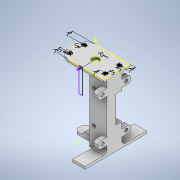
# Autodesk Inventor part: Gravitational viscometer P1
Saved by Autodesk Inventor 2020 (Build 240168000, 168)
## iProperties
Created: 2023-07-24
Part Number: Gravitational viscometer P1
Material: Generic
Document SubType Name: Modeling
Designer: 56992
Density: 1 g/cm^3
Appearance: Default
Author: 56992
Autodesk Inventor part; units mm, degrees
ref_plane "YZ Plane" through (0, 0, 0) normal (1, 0, 0) x (0, 1, 0)
ref_plane "XZ Plane" through (0, 0, 0) normal (0, 1, 0) x (-1, 0, 0)
ref_plane "XY Plane" through (0, 0, 0) normal (0, 0, 1) x (1, 0, 0)
sketch "Sketch1" plane through (0, 0, 0) normal (0, 0, 1) x (1, 0, 0)
  line L0 (0, 0) -> (30, 0)
  line L1 (30, 0) -> (30, 90)
  line L2 (30, 90) -> (0, 90)
  line L3 (0, 90) -> (0, 0)
  dimension "d0" = 90
  dimension "d1" = 30
  constraints: 8 end point, 2 parallel, 1 horizontal, 1 perpendicular
  measures "d0" distance between parallel lines of L0 L2
  measures "d1" distance between parallel lines of L3 L1
extrude "Extrusion1" add sketch "Sketch1" along normal blind 12
sketch "Sketch2" plane through (0, 90, 0) normal (0, 1, 0) x (1, 0, 0)
  circle A0 centre (6, -6) radius 3.9
  line L0 (30, 0) -> (0, 0) projected
  line L1 (0, 0) -> (0, -12) projected
  dimension "d4" = 7.8
  dimension "d5" = 6
  dimension "d6" = 6
  constraints: 1 centre point
  measures "d4" diameter of A0
  measures "d5" distance from line of L0 A0.centre
  measures "d6" distance from line of L1 A0.centre
extrude "Extrusion2" cut sketch "Sketch2" against normal blind 120
sketch "Sketch3" plane through (0, 0, 12) normal (0, 0, 1) x (1, 0, 0)
  line L0 (0, 90) -> (0, 0) projected
  line L1 (0, 83) -> (12, 83)
  line L2 (12, 83) -> (12, 7)
  line L3 (12, 7) -> (0, 7)
  line L4 (0, 7) -> (0, 83)
  line L5 (30, 90) -> (0, 90) projected
  line L6 (0, 0) -> (30, 0) projected
  point P0 (0, 7)
  dimension "d9" = 7
  dimension "d10" = 7
  dimension "d11" = 12
  constraints: 8 end point, 2 parallel, 1 horizontal, 1 perpendicular, 1 point on line
  measures "d9" distance between parallel lines of L5 L1
  measures "d10" distance between parallel lines of L6 L3
  measures "d11" distance between parallel lines of L0 L2
extrude "Extrusion3" cut sketch "Sketch3" against normal blind 120
sketch "Sketch4" plane through (0, 0, 0) normal (0, -1, 0) x (1, 0, 0)
  line L0 (30, 0) -> (30, 12) projected
  line L1 (30, 0) -> (0, 0)
  line L2 (0, 0) -> (0, -12)
  line L3 (0, -12) -> (30, -12)
  line L4 (30, -12) -> (30, 0)
  line L5 (0, 0) -> (0, 12) projected
  dimension "d14" = 0
  dimension "d15" = 12
  constraints: 8 end point, 2 parallel, 1 horizontal, 1 perpendicular
  measures "d14" distance between parallel lines of L5 L2
  measures "d15" distance between parallel lines of L1 L3
extrude "Extrusion4" add sketch "Sketch4" against normal blind 3
sketch "Sketch5" plane through (30, 90, 12) normal (0, 1, 0) x (1, 0, 0)
  point P0 (-30, 12)
sketch "Sketch6" plane through (0, 90, 0) normal (0, 1, 0) x (1, 0, 0)
  point P0 (0, 0)
sketch "Sketch7" plane through (30, 90, 12) normal (0, 1, 0) x (1, 0, 0)
  line L0 (-30, 0) -> (0, 0) projected
  line L1 (-30, 24) -> (-30, 0) projected
  line L2 (-10, 0) -> (-30, 0)
  line L3 (-30, 0) -> (-30, 24)
  line L4 (-30, 24) -> (-10, 24)
  line L5 (-10, 24) -> (-10, 0)
  circle A0 centre (-24, 6) radius 4.25 projected
  circle A1 centre (-24, 6) radius 3.75
  point P0 (-30, 12)
  point P1 (-25, 0)
  point P2 (-30, 5)
  point P3 (-30, 5)
  point P4 (-25, 0)
  dimension "d22" = 20
  dimension "d23" = 7.5
  constraints: 8 end point, 2 parallel, 1 centre point, 1 coincident, 1 horizontal, 1 perpendicular, 1 point on line
  measures "d22" distance between parallel lines of L1 L5
  measures "d23" diameter of A1
extrude "Extrusion5" add sketch "Sketch7" along normal blind 2 contours L1 L4 L5 L0 | A0
fillet "Fillet7" radius 0.5 4 edges at (2.25, 92, 6) (2.1, 83, 6) (2.1, 7, 6) (2.1, 0, 6)
chamfer "Chamfer2" distance 3 angle 45 1 edges at (10, 90, 0)
chamfer "Chamfer3" distance 3 angle 45 1 edges at (15, 3, 0)
chamfer "Chamfer4" [suppressed]
sketch "Sketch8" plane through (30, 92, 12) normal (0, 1, 0) x (1, 0, 0)
  point P0 (-30, 12)
sketch "Sketch9" plane through (30, 92, 12) normal (0, 1, 0) x (1, 0, 0)
  point P0 (-30, 12)
sketch "Sketch10" plane through (30, 92, 12) normal (0, 1, 0) x (1, 0, 0)
  line L0 (0, 12) -> (0, 0) projected
  line L1 (0, 12) -> (-30, 12)
  line L2 (-30, 12) -> (-30, 24)
  line L3 (-30, 24) -> (0, 24)
  line L4 (0, 24) -> (0, 12)
  line L5 (-30, 24) -> (-30, 0) projected
  line L6 (-10, 24) -> (-30, 24) projected
  point P0 (-30, 12)
  dimension "d41" = 0
  dimension "d42" = 0
  constraints: 8 end point, 2 parallel, 1 horizontal, 1 perpendicular
  measures "d41" distance between parallel lines of L5 L2
  measures "d42" distance between parallel lines of L6 L3
extrude "Extrusion6" cut sketch "Sketch10" against normal blind 100
sketch "Sketch11" plane through (0, 0, 0) normal (0, 0, -1) x (-1, 0, 0)
  line L0 (-19, 74) -> (-5.5, 74)
  line L1 (-5.5, 74) -> (-5.5, 8)
  line L2 (-5.5, 8) -> (-19, 8)
  line L3 (-19, 8) -> (-19, 74)
  line L4 (-12, 83) -> (0, 83) projected
  circle A0 centre (-15.3, 60) radius 2.05
  circle A1 centre (-15.3, 23) radius 2.05
  point P0 (0, 0)
  point P1 (0, 92)
  point P2 (-10, 83)
  dimension "d45" = 13.5
  dimension "d46" = 66
  dimension "d47" = 5.5
  dimension "d48" = 9
  dimension "d49" = 37
  dimension "d50" = 14
  dimension "d51" = 3.7
  dimension "d52" = 3.7
  dimension "d53" = 4.1
  dimension "d54" = 4.1
  constraints: 8 end point, 2 centre point, 2 parallel, 1 horizontal, 1 perpendicular
  measures "d45" distance between parallel lines of L1 L3
  measures "d46" distance between parallel lines of L2 L0
  measures "d47" distance from line of point (0, 92) L1
  measures "d48" distance between parallel lines of L4 L0
  measures "d49" distance of A1.centre A0.centre
  measures "d50" distance from line of L0 A0.centre
  measures "d51" distance from line of L3 A0.centre
  measures "d52" distance from line of L3 A1.centre
  measures "d53" diameter of A0
  measures "d54" diameter of A1
sketch "Sketch12" plane through (0, 0, 0) normal (0, 0, -1) x (-1, 0, 0)
  point P0 (0, 0)
extrude "Extrusion7" cut sketch "Sketch11" against normal blind 100 contours A0 | A1
sketch "Sketch13" plane through (0, 0, 0) normal (0, 0, -1) x (-1, 0, 0)
  line L0 (-10, 7) -> (-12, 9) projected
  line L1 (-10, 7) -> (-12, 7)
  line L2 (-12, 7) -> (-12, 83)
  line L3 (-12, 83) -> (-10, 83)
  line L4 (-10, 83) -> (-10, 7)
  line L5 (-12, 83) -> (0, 83) projected
  point P0 (0, 0)
  point P1 (-10, 83)
  dimension "d57" = 2
  dimension "d58" = 0
  constraints: 8 end point, 2 parallel, 1 horizontal, 1 perpendicular
  measures "d57" distance between parallel lines of L4 L2
  measures "d58" distance between parallel lines of L5 L3
extrude "Extrusion8" add sketch "Sketch13" against normal blind 12 contours L0 L2 L3 L4
sketch "Sketch14" plane through (0, 0, 0) normal (0, 0, -1) x (-1, 0, 0)
  line L0 (-15.3, 56.8) -> (-30, 56.8)
  line L1 (-30, 56.8) -> (-30, 26.2)
  line L2 (-30, 26.2) -> (-15.3, 26.2)
  line L3 (-15.3, 26.2) -> (-15.3, 56.8)
  circle A0 centre (-15.3, 60) radius 2.05 projected
  circle A1 centre (-15.3, 23) radius 2.05 projected
  line L4 (-30, 0) -> (-30, 90) projected
  line L5 (-10, 83) -> (0, 83) projected
  line L6 (-10, 83) -> (-15.3, 83)
  line L7 (-15.3, 83) -> (-15.3, 64)
  line L8 (-15.3, 64) -> (-10, 64)
  line L9 (-10, 64) -> (-10, 83)
  line L10 (-12, 9) -> (-10, 7) projected
  line L11 (-10, 7) -> (-15.3, 7)
  line L12 (-15.3, 7) -> (-15.3, 19)
  line L13 (-15.3, 19) -> (-10, 19)
  line L14 (-10, 19) -> (-10, 7)
  point P0 (0, 0)
  dimension "d61" = 3.2
  dimension "d62" = 3.2
  dimension "d63" = 0
  dimension "d64" = 0
  dimension "d67" = 0
  dimension "d68" = 4
  dimension "d69" = 4
  constraints: 24 end point, 6 parallel, 3 horizontal, 3 perpendicular, 1 point on line
  measures "d61" distance from line of A0.centre L0
  measures "d62" distance from line of A1.centre L2
  measures "d63" distance from line of A0.centre L3
  measures "d64" distance between parallel lines of L4 L1
  measures "d67" distance from line of A0.centre L7
  measures "d68" distance from line of A1.centre L13
  measures "d69" distance from line of A0.centre L8
extrude "Extrusion9" cut sketch "Sketch14" against normal blind 7 contours L3 L2 L1 L0
sketch "Sketch15" plane through (0, 0, 0) normal (0, 0, -1) x (-1, 0, 0)
  point P0 (0, 0)
extrude "Extrusion10" cut sketch "Sketch14" against normal blind 4 contours L9 L8 L7 L6 | L11 L12 L13 L14
sketch "Sketch16" plane through (0, 0, 12) normal (0, 0, 1) x (1, 0, 0)
  line L0 (30, 0) -> (30, 90) projected
  line L1 (0, 0) -> (30, 0) projected
  line L2 (30, 90) -> (10, 90)
  line L3 (10, 90) -> (10, 0)
  line L4 (10, 0) -> (30, 0)
  line L5 (30, 0) -> (30, 90)
  line L6 (10, 83) -> (10, 7) projected
  circle A0 centre (15.3, 60) radius 2.05 projected
  circle A1 centre (15.3, 60) radius 2.15
  circle A2 centre (15.3, 23) radius 2.05 projected
  circle A3 centre (15.3, 23) radius 2.15
  dimension "d72" = 0
  dimension "d73" = 4.1
  dimension "d74" = 37
  dimension "d75" = 5.3
  dimension "d76" = 23
  constraints: 8 end point, 2 centre point, 2 coincident, 2 parallel, 1 horizontal, 1 perpendicular, 1 point on line
  measures "d72" distance between parallel lines of L6 L3
  measures "d73" diameter of A0
  measures "d74" distance of A2.centre A0.centre
  measures "d75" distance from line of L3 A2.centre
  measures "d76" distance from line of L1 A2.centre
extrude "Extrusion11" add sketch "Sketch16" along normal blind 5 contours L1 L3 L2 L0 | A1 | A3
sketch "Sketch17" plane through (0, 0, 0) normal (0, -1, 0) x (1, 0, 0)
  line L0 (10, 17) -> (30, 17) projected
  line L1 (30, 17) -> (16, 17)
  line L2 (16, 17) -> (16, -18)
  line L3 (16, -18) -> (30, -18)
  line L4 (30, -18) -> (30, 17)
  point P0 (0, 0)
  point P1 (16, 17)
  dimension "d79" = 35
  dimension "d80" = 14
  constraints: 8 end point, 2 parallel, 1 horizontal, 1 perpendicular
  measures "d79" distance between parallel lines of L0 L3
  measures "d80" distance between parallel lines of L4 L2
extrude "Extrusion12" add sketch "Sketch17" against normal blind 3
sketch "Sketch18" plane through (0, 0, 0) normal (0, -1, 0) x (1, 0, 0)
  line L0 (30, 17) -> (16, 17)
  line L1 (16, 17) -> (16, 32)
  line L2 (16, 32) -> (30, 32)
  line L3 (30, 32) -> (30, 17)
  line L4 (0, 12) -> (10, 12) projected
  line L5 (16, 0) -> (16, -18) projected
  point P0 (0, 0)
  dimension "d83" = 20
  dimension "d84" = 0
  constraints: 8 end point, 2 parallel, 1 horizontal, 1 perpendicular
  measures "d83" distance between parallel lines of L4 L2
  measures "d84" distance between parallel lines of L5 L1
extrude "Extrusion13" add sketch "Sketch18" against normal blind 3
chamfer "Chamfer5" [suppressed]
sketch "Sketch19" plane through (20, 90, 0) normal (0, 1, 0) x (1, 0, 0)
  line L0 (-10, -12) -> (-10, -17) projected
  line L1 (10, 0) -> (10, -17) projected
  line L2 (-10, -17) -> (10, -17)
  line L3 (10, -17) -> (10, 0)
  line L4 (10, 0) -> (-10, 0)
  line L5 (-10, 0) -> (-10, -17)
  point P0 (-20, 0)
  constraints: 8 end point, 2 parallel, 1 horizontal, 1 perpendicular
extrude "Extrusion14" add sketch "Sketch19" along normal blind 2
sketch "Sketch20" plane through (30, 92, 12) normal (0, 1, 0) x (1, 0, 0)
  point P0 (-30, 12)
sketch "Sketch21" plane through (0, 83, 0) normal (-1, 0, 0) x (0, 0, 1)
  line L0 (0, -26.2) -> (0, 9) projected
  line L1 (12, 0) -> (12, 9) projected
  line L2 (0, 9) -> (12, 9)
  line L3 (12, 9) -> (12, 5)
  line L4 (12, 5) -> (0, 5)
  line L5 (0, 5) -> (0, 9)
  point P0 (0, -83)
  point P1 (0, 5)
  dimension "d92" = 4
  constraints: 8 end point, 2 parallel, 1 horizontal, 1 perpendicular, 1 point on line
  measures "d92" distance between parallel lines of L2 L4
extrude "Extrusion15" add sketch "Sketch21" along normal blind 5
sketch "Sketch22" plane through (30, 92, 12) normal (0, 1, 0) x (1, 0, 0)
  line L0 (-20, -5) -> (0, -5) projected
  line L1 (-35, 12) -> (-35, 0) projected
  line L2 (-20, -5) -> (-35, -5)
  line L3 (-35, -5) -> (-35, 0)
  line L4 (-35, 0) -> (-20, 0)
  line L5 (-20, 0) -> (-20, -5)
  point P0 (-30, 12)
  constraints: 8 end point, 2 parallel, 1 horizontal, 1 perpendicular
extrude "Extrusion16" add sketch "Sketch22" against normal blind 4
sketch "Sketch25" plane through (-5, 83, 0) normal (-1, 0, 0) x (0, 0, 1)
  line L0 (17, 9) -> (0, 9) projected
  line L1 (17, -80) -> (17, 9) projected
  line L2 (0, 9) -> (17, 9)
  line L3 (17, 9) -> (17, 5)
  line L4 (17, 5) -> (0, 5)
  line L5 (0, 5) -> (0, 9)
  line L6 (0, 5) -> (17, 5) projected
  line L7 (-2, 8) -> (19, 8)
  line L8 (19, 8) -> (19, 6)
  line L9 (19, 6) -> (-2, 6)
  line L10 (-2, 6) -> (-2, 8)
  point P0 (0, -83)
  dimension "d107" = 0
  dimension "d108" = 2
  dimension "d109" = 2
  dimension "d110" = 2
  dimension "d111" = 1
  dimension "d112" = 1
  constraints: 16 end point, 4 parallel, 2 horizontal, 2 perpendicular, 1 point on line
  measures "d107" distance between parallel lines of L6 L4
  measures "d108" distance between parallel lines of L9 L7
  measures "d109" distance between parallel lines of L1 L8
  measures "d110" distance between parallel lines of L5 L10
  measures "d111" distance between parallel lines of L0 L7
  measures "d112" distance between parallel lines of L4 L9
extrude "Extrusion17" add sketch "Sketch25" against normal blind 35 contours L7 L8 L9 L1 | L1 L9 L5 L7 | L5 L9 L10 L7
sketch "Sketch26" plane through (30, 92, 12) normal (0, 1, 0) x (1, 0, 0)
  arc A0 (-20, 7.4361) -> (-20, 4.5639) centre (-24, 6) ccw projected
  circle A1 centre (-24, 6) radius 3.9
  point P0 (-30, 12)
  dimension "d115" = 7.8
  constraints: 1 centre point, 1 coincident
  measures "d115" diameter of A1
extrude "Extrusion18" cut sketch "Sketch26" against normal blind 35
sketch "Sketch27" plane through (0, 0, 0) normal (-1, 0, 0) x (0, 0, 1)
  line L0 (12, 7) -> (12, 0) projected
  line L1 (0, 0) -> (12, 0)
  line L2 (12, 0) -> (12, 3)
  line L3 (12, 3) -> (0, 3)
  line L4 (0, 3) -> (0, 0)
  dimension "d118" = 3
  constraints: 8 end point, 2 parallel, 1 horizontal, 1 perpendicular, 1 point on line
  measures "d118" distance between parallel lines of L1 L3
extrude "Extrusion19" add sketch "Sketch27" along normal blind 6
chamfer "Chamfer6" distance 2 angle 45 2 edges at (-6, 1.5, 12) (-6, 1.5, 0)
fillet "Fillet8" radius 4 2 edges at (23, 3, 0) (23, 3, 17)
chamfer "Chamfer7" distance 4 angle 45 1 edges at (0, 3, 6)
sketch "Sketch28" plane through (-5, 89, -2) normal (0, 0, -1) x (-1, 0, 0)
  line L0 (0, 3) -> (-35, 3) projected
  line L1 (-35, 3) -> (0, 3)
  line L2 (0, 3) -> (0, -3)
  line L3 (0, -3) -> (-35, -3)
  line L4 (-35, -3) -> (-35, 3)
  line L5 (-20.3, -6) -> (-5, -6) projected
  point P0 (-5, -89)
  dimension "d128" = 3
  dimension "d129" = 5
  constraints: 8 end point, 2 parallel, 1 horizontal, 1 perpendicular
  measures "d128" distance between parallel lines of L5 L3
  measures "d129" distance from line of L5.end L2
extrude "Extrusion20" cut sketch "Sketch28" against normal blind 30
fillet_without_effect "Fillet9"
sketch "Sketch29" plane through (0, 83, 0) normal (0, -1, 0) x (1, 0, 0)
  point P0 (0, 0)
sketch "Sketch30" plane through (0, 0, 0) normal (0, 0, -1) x (-1, 0, 0)
  line L0 (-30, 7) -> (-30, 86) projected
  line L1 (-30, 86) -> (0, 86)
  line L2 (0, 86) -> (0, 76)
  line L3 (0, 76) -> (-30, 76)
  line L4 (-30, 76) -> (-30, 86)
  line L5 (-15.3, 83) -> (0, 83) projected
  point P0 (0, 0)
  dimension "d133" = 7
  dimension "d134" = 30
  constraints: 8 end point, 2 parallel, 1 horizontal, 1 perpendicular
  measures "d133" distance between parallel lines of L5 L3
  measures "d134" distance between parallel lines of L0 L2
extrude "Extrusion21" cut sketch "Sketch30" against normal blind 30
sketch "Sketch31" plane through (15.3, 76, 0) normal (0, 1, 0) x (1, 0, 0)
  line L0 (-2.05, 0) -> (2.05, 0) projected
  line L1 (-15.3, -12) -> (-15.3, 0) projected
  line L2 (0, 0) -> (-15.3, 0)
  line L3 (-15.3, 0) -> (-15.3, -12)
  line L4 (-15.3, -12) -> (0, -12)
  line L5 (0, -12) -> (0, 0)
  circle A0 centre (-9.3, -6) radius 3.9 projected
  circle A1 centre (-9.3, -6) radius 3.9
  line L6 (14.7, 0) -> (14.7, -17) projected
  line L7 (-5.3, -4) -> (-5.3, 0) projected
  line L8 (14.7, -17) -> (-5.3, -17)
  line L9 (-5.3, -17) -> (-5.3, 0)
  line L10 (-5.3, 0) -> (14.7, 0)
  line L11 (14.7, 0) -> (14.7, -17)
  point P0 (-15.3, 0)
  point P1 (-5.3, -12)
  point P2 (14.7, 0)
  point P3 (2.05, 0)
  point P4 (-2.05, 0)
  dimension "d137" = 7.8
  constraints: 16 end point, 4 parallel, 2 horizontal, 2 perpendicular, 1 centre point, 1 coincident, 1 midpoint
  measures "d137" diameter of A0
extrude "Extrusion22" add sketch "Sketch31" along normal blind 2
extrude "Extrusion23" add sketch "Sketch31" against normal blind 1
sketch "Sketch32" plane through (15.3, 78, 0) normal (0, 1, 0) x (1, 0, 0)
  point P0 (-15.3, 0)
sketch "Sketch33" plane through (15.3, 78, 0) normal (0, 1, 0) x (1, 0, 0)
  line L0 (-5.3, -12) -> (-15.3, -12)
  line L1 (-15.3, -12) -> (-15.3, -17)
  line L2 (-15.3, -17) -> (-5.3, -17)
  line L3 (-5.3, -17) -> (-5.3, -12)
  line L4 (-5.3, -17) -> (14.7, -17) projected
  line L5 (-15.3, 0) -> (-15.3, -12) projected
  dimension "d142" = 0
  dimension "d143" = 0
  constraints: 8 end point, 2 parallel, 1 horizontal, 1 perpendicular
  measures "d142" distance between parallel lines of L4 L2
  measures "d143" distance between parallel lines of L5 L1
extrude "Extrusion24" add sketch "Sketch33" against normal blind 3
sketch "Sketch34" plane through (0, 78, 0) normal (-1, 0, 0) x (0, 0, 1)
  line L0 (1.5, -0.5) -> (18.5, -0.5)
  line L1 (18.5, -0.5) -> (18.5, -2.5)
  line L2 (18.5, -2.5) -> (1.5, -2.5)
  line L3 (1.5, -2.5) -> (1.5, -0.5)
  line L4 (0, 0) -> (17, 0) projected
  line L5 (17, -3) -> (0, -3) projected
  line L6 (0, -3) -> (0, 0) projected
  line L7 (17, 0) -> (17, -3) projected
  point P0 (0, -78)
  point P1 (17, -0.5)
  point P2 (17, -2.5)
  point P3 (0, -2.5)
  point P4 (0, -0.5)
  dimension "d146" = 0.5
  dimension "d147" = 0.5
  dimension "d148" = 1.5
  dimension "d149" = 1.5
  constraints: 8 end point, 2 parallel, 1 horizontal, 1 perpendicular
  measures "d146" distance between parallel lines of L4 L0
  measures "d147" distance between parallel lines of L5 L2
  measures "d148" distance between parallel lines of L6 L3
  measures "d149" distance between parallel lines of L7 L1
fillet "Fillet10" radius 0.5 2 edges at (2.1, 78, 6) (2.1, 75, 6)
sketch "Sketch35" plane through (30, 26.2, 7) normal (1, 0, 0) x (0, 0, -1)
  line L0 (-20, 41.3) -> (17, 41.3)
  line L1 (17, 41.3) -> (17, 33.3)
  line L2 (17, 33.3) -> (-20, 33.3)
  line L3 (-20, 33.3) -> (-20, 41.3)
  line L4 (-20, -7.2) -> (17, -7.2)
  line L5 (17, -7.2) -> (17, -15.2)
  line L6 (17, -15.2) -> (-20, -15.2)
  line L7 (-20, -15.2) -> (-20, -7.2)
  line L8 (7, 30.6) -> (7, 51.8) projected
  line L9 (-10, -19.2) -> (-10, 51.8) projected
  line L10 (-25, -23.2) -> (-14, -23.2) projected
  line L11 (-11.5, 49.3) -> (-10, 49.3) projected
  point P0 (7, -26.2)
  point P1 (7, 49.3)
  dimension "d153" = 10
  dimension "d154" = 10
  dimension "d155" = 8
  dimension "d156" = 8
  dimension "d157" = 8
  dimension "d158" = 8
  constraints: 16 end point, 4 parallel, 2 horizontal, 2 perpendicular, 2 point on line
  measures "d153" distance between parallel lines of L8 L1
  measures "d154" distance between parallel lines of L9 L3
  measures "d155" distance between parallel lines of L2 L0
  measures "d156" distance between parallel lines of L6 L4
  measures "d157" distance between parallel lines of L10 L6
  measures "d158" distance between parallel lines of L11 L0
extrude "Extrusion26" add sketch "Sketch35" against normal blind 5
sketch "Sketch36" plane through (30, 26.2, 7) normal (1, 0, 0) x (0, 0, -1)
  circle A0 centre (-15, 37.3) radius 1.6
  circle A1 centre (12, 37.3) radius 1.6
  circle A2 centre (-15, -11.2) radius 1.6
  circle A3 centre (12, -11.2) radius 1.6
  line L0 (-10, -7.2) -> (-10, 33.3) projected
  line L1 (7, 30.6) -> (7, 33.3) projected
  line L2 (7, -7.2) -> (7, 0) projected
  line L3 (-20, -15.2) -> (-10, -15.2) projected
  line L4 (7, -15.2) -> (17, -15.2) projected
  line L5 (7, 33.3) -> (17, 33.3) projected
  line L6 (-20, 33.3) -> (-10, 33.3) projected
  point P0 (7, -26.2)
  dimension "d161" = 5
  dimension "d162" = 5
  dimension "d163" = 5
  dimension "d164" = 5
  dimension "d165" = 4
  dimension "d166" = 4
  dimension "d167" = 4
  dimension "d168" = 4
  dimension "d169" = 3.2
  dimension "d170" = 3.2
  dimension "d171" = 3.2
  dimension "d172" = 3.2
  constraints: 4 centre point
  measures "d161" distance from line of L0 A0.centre
  measures "d162" distance from line of L1 A1.centre
  measures "d163" distance from line of L2 A3.centre
  measures "d164" distance from line of L0 A2.centre
  measures "d165" distance from line of L3 A2.centre
  measures "d166" distance from line of L4 A3.centre
  measures "d167" distance from line of L5 A1.centre
  measures "d168" distance from line of L6 A0.centre
  measures "d169" diameter of A0
  measures "d170" diameter of A1
  measures "d171" diameter of A3
  measures "d172" diameter of A2
extrude "Extrusion27" cut sketch "Sketch36" against normal blind 6
fillet "Fillet12" radius 3 8 edges at (27.5, 67.5, 27) (27.5, 59.5, 27) (27.5, 19, 27) (27.5, 11, 27) (27.5, 67.5, -10) (27.5, 19, -10) (27.5, 11, -10) (27.5, 59.5, -10)
sketch "Sketch37" plane through (0, 0, 4) normal (0, 0, -1) x (-1, 0, 0)
  line L0 (-10, 7) -> (-12, 9) projected
  line L1 (-10, 7) -> (-12, 7)
  line L2 (-12, 7) -> (-12, 10)
  line L3 (-12, 10) -> (-10, 10)
  line L4 (-10, 10) -> (-10, 7)
  line L5 (-12, 9) -> (-12, 7) projected
  point P0 (0, 0)
  dimension "d177" = 0
  dimension "d178" = 3
  constraints: 8 end point, 2 parallel, 1 horizontal, 1 perpendicular
  measures "d177" distance between parallel lines of L5 L2
  measures "d178" distance between parallel lines of L1 L3
extrude "Extrusion28" add sketch "Sketch37" against normal blind 13
sketch "Sketch38" plane through (0, 0, 0) normal (0, 0, -1) x (-1, 0, 0)
  line L0 (-15.3, 56.8) -> (-15.3, 26.2) projected
  line L1 (-15.3, 54.8) -> (-12.3, 54.8)
  line L2 (-12.3, 54.8) -> (-12.3, 28.2)
  line L3 (-12.3, 28.2) -> (-15.3, 28.2)
  line L4 (-15.3, 28.2) -> (-15.3, 54.8)
  line L5 (-30, 56.8) -> (-15.3, 56.8) projected
  line L6 (-15.3, 26.2) -> (-30, 26.2) projected
  point P0 (0, 0)
  dimension "d181" = 3
  dimension "d182" = 2
  dimension "d183" = 2
  constraints: 8 end point, 2 parallel, 1 horizontal, 1 perpendicular, 1 point on line
  measures "d181" distance between parallel lines of L0 L2
  measures "d182" distance between parallel lines of L5 L1
  measures "d183" distance between parallel lines of L6 L3
extrude "Extrusion29" cut sketch "Sketch38" against normal blind 4
sketch "Sketch39" plane through (15.3, 78, 0) normal (0, 1, 0) x (1, 0, 0)
  line L0 (-15.3, -17) -> (14.7, -17) projected
  line L1 (14.7, -17) -> (-35.3, -17)
  line L2 (-35.3, -17) -> (-35.3, -21)
  line L3 (-35.3, -21) -> (14.7, -21)
  line L4 (14.7, -21) -> (14.7, -17)
  line L5 (-15.3, 0) -> (-15.3, -17) projected
  line L6 (14.7, 0) -> (14.7, -7) projected
  line L7 (14.7, 0) -> (-35.3, 0)
  line L8 (-35.3, 0) -> (-35.3, 9)
  line L9 (-35.3, 9) -> (14.7, 9)
  line L10 (14.7, 9) -> (14.7, 0)
  circle A0 centre (-9.3, -6) radius 3.9 projected
  line L11 (-15.3, -17) -> (-15.3, 0) projected
  line L12 (-35.3, -21) -> (-15.3, -21)
  line L13 (-15.3, -21) -> (-15.3, 0)
  line L14 (-15.3, 0) -> (-35.3, 0)
  line L15 (-35.3, 0) -> (-35.3, -21)
  point P0 (-15.3, 0)
  dimension "d186" = 20
  dimension "d187" = 4
  dimension "d188" = 15
  dimension "d189" = 0
  constraints: 24 end point, 6 parallel, 3 horizontal, 3 perpendicular
  measures "d186" distance between parallel lines of L2 L5
  measures "d187" distance between parallel lines of L0 L3
  measures "d188" distance from line of A0.centre L9
  measures "d189" distance between parallel lines of L2 L8
extrude "Extrusion30" add sketch "Sketch39" against normal blind 3 contours L13 L3 L2 L1 | L1 L15 L7 L5 | L0 L4 L3 L13 | L7 L8 L9 L10
fillet "Fillet13" radius 10 2 edges at (-20, 76.5, -9) (-20, 76.5, 21)
sketch "Sketch40" plane through (10, 0, 12) normal (0, -1, 0) x (1, 0, 0)
  line L0 (6, 20) -> (20, 20) projected
  line L1 (6, 20) -> (20, 20)
  line L2 (20, 20) -> (20, 30)
  line L3 (20, 30) -> (6, 30)
  line L4 (6, 30) -> (6, 20)
  line L5 (6, -30) -> (20, -30) projected
  line L6 (20, -30) -> (6, -30)
  line L7 (6, -30) -> (6, -40)
  line L8 (6, -40) -> (20, -40)
  line L9 (20, -40) -> (20, -30)
  line L10 (6, 20) -> (6, 5) projected
  point P0 (-10, -12)
  dimension "d193" = 10
  dimension "d194" = 10
  dimension "d195" = 14
  constraints: 16 end point, 4 parallel, 2 horizontal, 2 perpendicular, 1 point on line
  measures "d193" distance between parallel lines of L5 L8
  measures "d194" distance between parallel lines of L0 L3
  measures "d195" distance between parallel lines of L10 L2
extrude "Extrusion31" add sketch "Sketch40" against normal blind 3
sketch "Sketch41" plane through (10, 0, 12) normal (0, -1, 0) x (1, 0, 0)
  line L0 (-14, -12) -> (-14, 0) projected
  line L1 (-14, -12) -> (-22, -12)
  line L2 (-22, -12) -> (-22, 0)
  line L3 (-22, 0) -> (-14, 0)
  line L4 (-14, 0) -> (-14, -12)
  point P0 (-10, -12)
  dimension "d198" = 8
  dimension "d199" = 12
  constraints: 8 end point, 2 parallel, 1 horizontal, 1 perpendicular
  measures "d198" distance between parallel lines of L0 L2
  measures "d199" distance between parallel lines of L1 L3
extrude "Extrusion32" add sketch "Sketch41" against normal blind 3
chamfer "Chamfer8" distance 3 angle 45 2 edges at (-12, 1.5, 12) (-12, 1.5, 0)
fillet "Fillet14" radius 0.4 4 edges at (30, 63.5, 23.6) (30, 63.5, -3.4) (30, 15, -3.4) (30, 15, 23.6)
chamfer "Chamfer9" distance 2 angle 45 4 edges at (25, 63.5, 23.6) (25, 15, 23.6) (25, 63.5, -3.4) (25, 15, -3.4)
sketch "Sketch42" plane through (10, 0, 12) normal (0, -1, 0) x (1, 0, 0)
  arc A0 (0, -4.167) -> (0, -7.833) centre (-4, -6) ccw projected
  circle A1 centre (-4, -6) radius 4.4
  line L0 (-22, -3) -> (-22, -9) projected
  line L1 (0, 0) -> (-19, 0) projected
  point P0 (-10, -12)
  point P1 (0, -7.833)
  dimension "d209" = 4.4
  dimension "d210" = 18
  dimension "d211" = 6
  constraints: 1 centre point, 1 coincident
  measures "d209" radius of A0
  measures "d210" distance from line of L0 A0.centre
  measures "d211" distance from line of L1 A0.centre
extrude "Extrusion33" add sketch "Sketch42" against normal blind 2
sketch "Sketch43" plane through (15.3, 78, 0) normal (0, 1, 0) x (1, 0, 0)
  circle A0 centre (-30.3, 2) radius 2
  circle A1 centre (-30.3, -14) radius 2
  circle A2 centre (9.7, 2) radius 2
  circle A3 centre (9.7, -14) radius 2
  line L0 (-35.3, -1) -> (-35.3, -11) projected
  line L1 (-25.3, -21) -> (14.7, -21) projected
  line L2 (14.7, 9) -> (-25.3, 9) projected
  line L3 (14.7, -21) -> (14.7, 9) projected
  point P0 (-15.3, 0)
  dimension "d214" = 5
  dimension "d215" = 7
  dimension "d216" = 5
  dimension "d217" = 7
  dimension "d218" = 5
  dimension "d219" = 7
  dimension "d220" = 7
  dimension "d221" = 5
  dimension "d222" = 4
  dimension "d223" = 4
  dimension "d224" = 4
  dimension "d225" = 4
  constraints: 4 centre point
  measures "d214" distance from line of L0 A1.centre
  measures "d215" distance from line of L1 A1.centre
  measures "d216" distance from line of L0 A0.centre
  measures "d217" distance from line of L2 A0.centre
  measures "d218" distance from line of L3 A2.centre
  measures "d219" distance from line of L2 A2.centre
  measures "d220" distance from line of L1 A3.centre
  measures "d221" distance from line of L3 A3.centre
  measures "d222" diameter of A3
  measures "d223" diameter of A2
  measures "d224" diameter of A1
  measures "d225" diameter of A0
extrude "Extrusion34" cut sketch "Sketch43" against normal blind 3
sketch "Sketch44" plane through (6, 2, 6) normal (0, 1, 0) x (1, 0, 0)
  circle A0 centre (0, 0) radius 3.9 projected
  circle A1 centre (0, 0) radius 1.7
  point P0 (-6, 6)
  dimension "d228" = 3.4
  constraints: 1 centre point, 1 coincident
  measures "d228" diameter of A1
extrude "Extrusion35" cut sketch "Sketch44" against normal blind 3 contours A1
sketch "Sketch45" plane through (15.3, 78, 0) normal (0, 1, 0) x (1, 0, 0)
  point P0 (-15.3, 0)
sketch "Sketch46" plane through (15.3, 78, 0) normal (0, 1, 0) x (1, 0, 0)
  line L0 (14.7, -21) -> (-25.3, -21) projected
  line L1 (-10.4513, -21) -> (-9.3, -21)
  line L2 (-9.3, -21) -> (-9.3, -26.3856)
  line L3 (-9.3, -26.3856) -> (-10.4513, -26.3856)
  line L4 (-10.4513, -26.3856) -> (-10.4513, -21)
  circle A0 centre (-9.3, -6) radius 4.4 projected
  point P0 (-15.3, 0)
  dimension "d231" = 0
  constraints: 8 end point, 2 parallel, 1 horizontal, 1 perpendicular, 1 point on line
  measures "d231" distance from line of A0.centre L2
sketch "Sketch47" plane through (30, 75, 21) normal (0, 0, 1) x (1, 0, 0)
  line L0 (-19.6, 3) -> (-28.4, 3) projected
  line L1 (-24, 3) -> (-27.9039, 3)
  line L2 (-27.9039, 3) -> (-27.9039, -24.6997)
  line L3 (-27.9039, -24.6997) -> (-24, -24.6997)
  line L4 (-24, -24.6997) -> (-24, 3)
  point P0 (-30, -75)
  constraints: 8 end point, 2 parallel, 1 horizontal, 1 midpoint, 1 perpendicular
body "Solid1"
